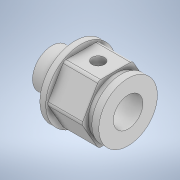
# Autodesk Inventor part: banebot_hubs_small_1_4
Saved by Autodesk Inventor 2020 (Build 240168000, 168)
## iProperties
Created: 2020-02-10
Part Number: banebot_hubs_small_1_4
Material: Generic
Document SubType Name: Modeling
Designer: akend
Density: 1 g/cm^3
Appearance: Default
Author: akend
## iProperties of the stored document _3DPrint.ipt
Created: 2020-02-10
Part Number: _3DPrint
Material: Generic
Document SubType Name: Modeling
Designer: akend
Density: 1 g/cm^3
Appearance: Default
Author: akend
Autodesk Inventor part; units mm, degrees
ref_plane "YZ Plane" through (0, 0, 0) normal (1, 0, 0) x (0, 1, 0)
ref_plane "XZ Plane" through (0, 0, 0) normal (0, 1, 0) x (-1, 0, 0)
ref_plane "XY Plane" through (0, 0, 0) normal (0, 0, 1) x (1, 0, 0)
sketch "Sketch1" plane through (0, 0, 0) normal (1, 0, 0) x (0, 1, 0)
  circle A0 centre (0, 0) radius 7.5985
  dimension "d0" = 15.197
  constraints: 1 centre point, 1 coincident
  measures "d0" diameter of A0
extrude "Extrusion1" add sketch "Sketch1" along normal blind 1.28
sketch "Sketch2" plane through (1.28, 0, 0) normal (1, 0, 0) x (0, 0, -1)
  line L0 (3.6604, 6.34) -> (7.3208, 0)
  line L1 (7.3208, 0) -> (3.6604, -6.34)
  line L2 (3.6604, -6.34) -> (-3.6604, -6.34)
  line L3 (-3.6604, -6.34) -> (-7.3208, 0)
  line L4 (-7.3208, 0) -> (-3.6604, 6.34)
  line L5 (-3.6604, 6.34) -> (3.6604, 6.34)
  point P0 (0, 0)
  point P1 (0, 6.34)
  point P2 (0, 0)
  constraints: 12 end point, 1 coincident, 1 midpoint, 13 other
extrude "Extrusion2" add sketch "Sketch2" along normal blind 7.5
sketch "Sketch3" plane through (8.78, 0, 0) normal (1, 0, 0) x (0, 0, -1)
  circle A0 centre (0, 0) radius 5.927
  dimension "d5" = 11.854
  constraints: 1 centre point, 1 coincident
  measures "d5" diameter of A0
extrude "Extrusion3" add sketch "Sketch3" along normal blind 1.22
sketch "Sketch4" plane through (10, 0, 0) normal (1, 0, 0) x (0, 0, -1)
  circle A0 centre (0, 0) radius 6.34
  line L0 (3.6604, 6.34) -> (-3.6604, 6.34) projected
  constraints: 1 centre point, 1 coincident, 1 tangent
extrude "Extrusion4" add sketch "Sketch4" along normal blind 1.5
fillet "Fillet1" radius 0.75 5 edges at (5.03, 0, -7.3208) (5.03, -6.34, -3.6604) (5.03, 0, 7.3208) (5.03, 6.34, -3.6604) (5.03, 6.34, 3.6604)
fillet "Fillet2" radius 0.75 1 edges at (5.03, -6.34, 3.6604)
sketch "Sketch5" plane through (0, 0, 0) normal (-1, 0, 0) x (0, 0, 1)
  point P0 (0, 0)
sketch "Sketch6" plane through (1.28, 6.34, 3.2274) normal (0, 1, 0) x (1, 0, 0)
  circle A0 centre (3.75, 3.2274) radius 1.3525
  point P0 (-1.28, 3.2274)
  dimension "d12" = 2.705
  constraints: 1 centre point, 1 coincident
  measures "d12" diameter of A0
extrude "Extrusion5" cut sketch "Sketch6" against normal blind 6.5
sketch "Sketch7" plane through (0, 0, 0) normal (-1, 0, 0) x (0, 0, 1)
  circle A0 centre (0, 0) radius 3.2
  dimension "d15" = 6.4
  constraints: 1 centre point, 1 coincident
  measures "d15" diameter of A0
sketch "Sketch8" plane through (5.03, -0.16, 0) normal (0, 1, 0) x (1, 0, 0)
  point P0 (-5.03, 0)
extrude "Extrusion6" cut sketch "Sketch7" against normal blind 11.75
sketch "Sketch9" plane through (0, 0, 0) normal (-1, 0, 0) x (0, 0, 1)
  circle A0 centre (0, 0) radius 3.2
  circle A1 centre (0, 0) radius 4.2
  dimension "d18" = 8.4
  constraints: 2 centre point, 2 coincident
  measures "d18" diameter of A1
extrude "Extrusion7" add sketch "Sketch9" along normal blind 5
fillet "Fillet3" radius 2 1 edges at (0, 0, -4.2)
body "Solid1"
